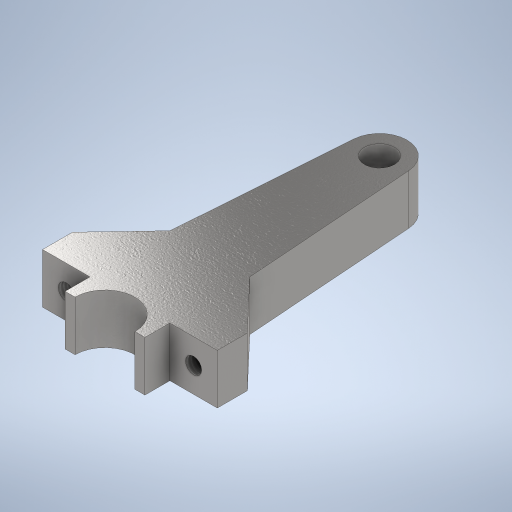
# Autodesk Inventor part: Pleuel_oberteil
Saved by Autodesk Inventor 2024 (Build 280153000, 153)
## iProperties
Created: 2024-02-29
Part Number: Pleuel_oberteil
Material: Stahl, galvanisiert
Document SubType Name: Modeling
Designer: ffogue
Density: 7.85 g/cm^3
Appearance: Galvanisiert
Author: ffogue
Autodesk Inventor part; units mm, degrees
ref_plane "YZ Plane" through (0, 0, 0) normal (1, 0, 0) x (0, 1, 0)
ref_plane "XZ Plane" through (0, 0, 0) normal (0, 1, 0) x (-1, 0, 0)
ref_plane "XY Plane" through (0, 0, 0) normal (0, 0, 1) x (1, 0, 0)
sketch "Skizze1" plane through (0, 0, 0) normal (0, 0, 1) x (1, 0, 0)
  line L0 (0, 0) -> (0, 60.5) construction
  line L1 (0, 0) -> (-8, 0)
  line L2 (-8, 0) -> (-8, 5)
  line L3 (-8, 5) -> (-17.5, 5)
  line L4 (-17.5, 5) -> (-17.5, 11)
  line L5 (-17.5, 11) -> (-8, 21)
  line L6 (-8, 21) -> (-5.5, 55.3854)
  arc A0 (5.5, 55.3854) -> (-5.5, 55.3854) centre (0, 54.9855) ccw
  line L7 (5.5, 55.3854) -> (8, 21)
  line L8 (8, 21) -> (17.5, 11)
  line L9 (17.5, 11) -> (17.5, 5)
  line L10 (17.5, 5) -> (8, 5)
  line L11 (8, 5) -> (8, 0)
  line L12 (8, 0) -> (0, 0)
  dimension "d6" = 60.5
  dimension "d7" = 16
  dimension "d8" = 5
  dimension "d9" = 11
  dimension "d10" = 35
  dimension "d11" = 11
  dimension "d12" = 21
  constraints: 26 end point, 6 perpendicular, 3 point on circle, 2 parallel, 2 symmetric about line, 2 vertical, 1 centre point, 1 coincident, 1 horizontal, 1 point on line, 1 tangent, 1 vertical alignment, 2 other
  measures "d6" distance of L0.end L0.start
  measures "d7" distance between parallel lines of L11 L2
  measures "d8" distance between parallel lines of L12 L10
  measures "d9" distance of L7.start L6.end
  measures "d10" distance between parallel lines of L9 L4
  measures "d11" distance from line of L12 L8.end
  measures "d12" distance from line of L12 L7.end
extrude "Extrusion1" add sketch "Skizze1" along normal blind 10
sketch "Skizze2" plane through (0, 0, 10) normal (0, 0, 1) x (1, 0, 0)
  line L0 (-8, 0) -> (8, 0) projected
  arc A0 (6, 0) -> (-6, 0) centre (0, 0) ccw
  point P0 (0, 0)
  dimension "d15" = 12
  constraints: 2 coincident, 2 midpoint, 2 point on circle, 2 point on line, 1 centre point
  measures "d15" distance of A0.start A0.end
extrude "Extrusion2" cut sketch "Skizze2" against normal blind 10
sketch "Skizze3" plane through (-17.5, 5, 0) normal (0, -1, 0) x (1, 0, 0)
  line L0 (17.5, 0) -> (17.5, 10) construction
  line L1 (11.5, 10) -> (23.5, 10) projected
  line L2 (0, 0) -> (0, 10) projected
  point P0 (4.75, 5)
  point P1 (30.25, 5)
  point P2 (0, 5)
  dimension "d18" = 25.5
  constraints: 2 end point, 2 midpoint, 1 horizontal alignment, 1 symmetric about line
  measures "d18" distance of point (30.25, 5) point (4.75, 5)
hole "Bohrung1" at (-12.75, 5, 5) at (12.75, 5, 5) direction (0, 1, 0) diameter 3.242 depth 9 tip angle 118 thread size "M4x0.7" class "6H" standard "ISO Metric profile"
sketch "Skizze4" plane through (0, 0, 10) normal (0, 0, 1) x (1, 0, 0)
  arc A0 (5.5, 55.3854) -> (-5.5, 55.3854) centre (0, 54.9855) ccw projected
  point P0 (0, 0)
  constraints: 1 coincident
hole "Bohrung2" at (0, 54.9855, 10) direction (0, 0, -1) diameter 6.02 end through all
